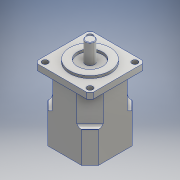
# Autodesk Inventor part: N2-0028-30-24
Saved by Autodesk Inventor 2016 SP1 (Build 200210100, 210)
## iProperties
Created: 2018-06-12
Part Number: N2-0028-30-24
Material: Aluminium 6061
Document SubType Name: Modeling
Designer: dimercur
Mass: 49.005 g
Surface Area: 73.7 cm^2
Volume: 18.15 cm^3
Density: 2.7 g/cm^3
Appearance: Aluminium - Plat
Author: dimercur
Autodesk Inventor part; units mm, degrees
ref_plane "YZ Plane" through (0, 0, 0) normal (1, 0, 0) x (0, 1, 0)
ref_plane "XZ Plane" through (0, 0, 0) normal (0, 1, 0) x (-1, 0, 0)
ref_plane "XY Plane" through (0, 0, 0) normal (0, 0, 1) x (1, 0, 0)
sketch "Esquisse1" plane through (0, 0, 0) normal (0, 0, 1) x (1, 0, 0)
  line L0 (-25, 25) -> (25, 25)
  line L1 (25, 25) -> (25, -25)
  line L2 (25, -25) -> (-25, -25)
  line L3 (-25, -25) -> (-25, 25)
  point P0 (0, 0)
  dimension "d0" = 50
  dimension "d1" = 25
  dimension "d2" = 50
  dimension "d3" = 25
  constraints: 8 end point, 2 parallel, 1 horizontal, 1 perpendicular
  measures "d0" distance of L0.end L0.start
  measures "d1" horizontal distance of point (0, 0) L0.start
  measures "d2" distance of L2.end L0.start
  measures "d3" horizontal distance of point (0, 0) L0.start
extrude "Extrusion1" add sketch "Esquisse1" along normal blind 31
chamfer "Chanfrein1" distance 8 angle 45 4 edges at (25, 25, 15.5) (-25, 25, 15.5) (-25, -25, 15.5) (25, -25, 15.5)
sketch "Esquisse4" plane through (0, 0, 31) normal (0, 0, 1) x (1, 0, 0)
  line L0 (17, 25) -> (-17, 25) projected
  line L1 (-12, 25) -> (12, 25)
  line L2 (25, 17) -> (25, -17) projected
  line L3 (25, 12) -> (25, -12)
  line L4 (-17, -25) -> (17, -25) projected
  line L5 (12, -25) -> (-12, -25)
  line L6 (-25, 17) -> (-25, -17) projected
  line L7 (-25, -12) -> (-25, 12)
  line L8 (-25, 12) -> (-12, 25)
  line L9 (12, 25) -> (25, 12)
  line L10 (17, 25) -> (25, 17) projected
  line L11 (25, -12) -> (12, -25)
  line L12 (-12, -25) -> (-25, -12)
  point P0 (0, 0)
  dimension "d11" = 24
  dimension "d12" = 24
  dimension "d13" = 24
  dimension "d14" = 24
  dimension "d15" = 12
  dimension "d16" = 12
  constraints: 16 end point, 8 point on line, 1 parallel, 1 perpendicular
  measures "d11" distance of L7.end L7.start
  measures "d12" distance of L1.end L1.start
  measures "d13" distance of L3.end L3.start
  measures "d14" distance of L5.start L5.end
  measures "d15" horizontal distance of point (0, 0) L5.end
  measures "d16" vertical distance of point (0, 0) L7.end
extrude "Extrusion3" add sketch "Esquisse4" along normal blind 31 contours L9 L2 L11 L4 L12 L6 L8 L0
sketch "Esquisse5" plane through (0, 0, 62) normal (0, 0, 1) x (1, 0, 0)
  line L0 (-27.5, 27.5) -> (27.5, 27.5)
  line L1 (27.5, 27.5) -> (27.5, -27.5)
  line L2 (27.5, -27.5) -> (-27.5, -27.5)
  line L3 (-27.5, -27.5) -> (-27.5, 27.5)
  point P0 (0, 0)
  dimension "d19" = 55
  dimension "d20" = 55
  dimension "d21" = 27.5
  dimension "d22" = 27.5
  constraints: 8 end point, 2 parallel, 1 horizontal, 1 perpendicular
  measures "d19" distance of L0.start L0.end
  measures "d20" distance of L2.end L0.start
  measures "d21" horizontal distance of point (0, 0) L0.start
  measures "d22" horizontal distance of point (0, 0) L0.start
extrude "Extrusion4" add sketch "Esquisse5" along normal blind 6
sketch "Esquisse6" plane through (0, 0, 68) normal (0, 0, 1) x (1, 0, 0)
  circle A0 centre (0, 0) radius 20
  circle A1 centre (0, 0) radius 12.5
  dimension "d25" = 40
  dimension "d26" = 25
  constraints: 2 centre point, 2 coincident
  measures "d25" diameter of A0
  measures "d26" diameter of A1
extrude "Extrusion5" add sketch "Esquisse6" along normal blind 2.5
sketch "Esquisse7" plane through (0, 0, 68) normal (0, 0, 1) x (1, 0, 0)
  circle A0 centre (0, 0) radius 4.5
  dimension "d29" = 9
  constraints: 1 centre point, 1 coincident
  measures "d29" diameter of A0
extrude "Extrusion6" add sketch "Esquisse7" along normal blind 20
sketch "Esquisse8" plane through (0, 0, 68) normal (0, 0, 1) x (1, 0, 0)
  circle A0 centre (-22.2739, 22.2739) radius 2.9
  line L0 (-22.2739, 22.2739) -> (-27.5, 22.2739)
  line L1 (-27.5, 27.5) -> (-27.5, -27.5) projected
  line L2 (-22.2739, 22.2739) -> (-22.2739, 27.5)
  line L3 (27.5, 27.5) -> (-27.5, 27.5) projected
  circle A1 centre (-22.2739, -22.2739) radius 2.9
  circle A2 centre (22.2739, -22.2739) radius 2.9
  circle A3 centre (22.2739, 22.2739) radius 2.9
  point P0 (0, 0)
  dimension "d32" = 5.8
  dimension "d33" = 31.5
  dimension "d36" = 360
  constraints: 4 centre point, 4 end point, 2 perpendicular, 2 point on line, 1 horizontal, 9 other
  measures "d32" diameter of A0
  measures "d33" distance of point (0, 0) L0.start
extrude "Extrusion7" cut sketch "Esquisse8" against normal blind 6 contours A0 L0 L2 | L2 L0 A0 | A1 | A2 | A3
chamfer "Chanfrein2" distance 3 angle 45 4 edges at (-27.5, 27.5, 65) (27.5, 27.5, 65) (27.5, -27.5, 65) (-27.5, -27.5, 65)
fillet "Congé1" radius 3 4 edges at (18.5, 18.5, 31) (18.5, -18.5, 31) (-18.5, 18.5, 31) (-18.5, -18.5, 31)
chamfer "Chanfrein3" distance 0.5 angle 45 1 edges at (-4.5, 0, 88)
equation "\"d1\" = 0.5 * d0"
equation "\"d2\" = d0"
equation "\"d3\" = 0.5 * d2"
equation "\"d12\" = d11"
equation "\"d13\" = d11"
equation "\"d14\" = d11"
equation "\"d15\" = 0.5 * d14"
equation "\"d16\" = 0.5 * d11"
equation "\"d20\" = d19"
equation "\"d21\" = 0.5 * d20"
equation "\"d22\" = 0.5 * d19"
